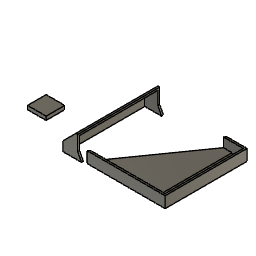
newest fin air guid v5 (Autodesk Fusion 360 design; units mm, degrees)
Autodesk Fusion 360 part; units mm, degrees
sketch "Sketch1" plane through (0, 0, 0) normal (0, 0, 1) x (1, 0, 0)
  line L0 (0, 0) -> (42, 0)
  line L1 (42, 0) -> (42, 44)
  line L2 (42, 44) -> (31, 44)
  line L3 (31, 44) -> (0, 0)
  dimension "d1" = 42
  dimension "d2" = 44
  dimension "d3" = 11
  constraint coincident L0.start L3.end
  constraint horizontal L0
  constraint perpendicular L0 L1
  constraint perpendicular L1 L2
  measures "d1" distance of L0.start L0.end
  measures "d2" distance of L0.end L1.end
  measures "d3" distance of L1.end L2.end
extrude "Extrude1" add sketch "Sketch1" along normal blind 6 makes body 1
sketch "Sketch2" plane through (42, 0, 0) normal (1, 0, 0) x (0, 1, 0)
  line L0 (0, 0) -> (44, 0)
  line L1 (44, 0) -> (44, 6)
  line L2 (44, 6) -> (0, 6)
  line L3 (0, 6) -> (0, 0)
  line L4 (1, 5) -> (43, 5)
  line L5 (43, 5) -> (43, 0)
  line L6 (43, 0) -> (1, 0)
  line L7 (1, 0) -> (1, 5)
  constraint horizontal L4
  constraint vertical L5
  constraint horizontal L6
  constraint vertical L7
  constraint coincident L0 L5.end
extrude "Extrude2" cut sketch "Sketch2" against normal blind 70 contours L0 L4 L5 L6 L7 bodies 1
sketch "Sketch3" plane through (0, 0, 5) normal (0, 0, -1) x (1, 0, 0)
  line L0 (0.7045, -1) -> (30.2955, -43)
  line L1 (30.2955, -43) -> (42, -43)
  line L2 (42, -43) -> (42, -1)
  line L3 (42, -1) -> (0.7045, -1)
  line L4 (42, -43) -> (41, -43)
  line L5 (41, -43) -> (41, -1)
  line L6 (41, -1) -> (42, -1)
  line L7 (42, -1) -> (42, -43)
  constraint horizontal L4
  constraint vertical L5
  constraint horizontal L6
  constraint vertical L7
  constraint coincident L3 L5.end
  constraint coincident L1.end L2.start
extrude "Extrude3" add sketch "Sketch3" along normal blind 5 contours L1 L2 L3 L4 L5 L6 L7 bodies 1
sketch "Sketch4" plane through (0, 0, 5) normal (0, 0, -1) x (1, 0, 0)
  line L0 (41, -43) -> (41, -1)
  line L1 (41, -1) -> (0.7045, -1)
  line L2 (0.7045, -1) -> (30.2955, -43)
  line L3 (30.2955, -43) -> (41, -43)
  line L4 (41, -43) -> (35, -43)
  line L5 (35, -43) -> (35, -1)
  line L6 (35, -1) -> (41, -1)
  line L7 (41, -1) -> (41, -43)
  dimension "d10" = 6
  dimension "d11" = 42
  constraint horizontal L4
  constraint vertical L5
  constraint horizontal L6
  constraint vertical L7
  constraint coincident L0.start L3.end
  measures "d10" distance of L0.start L4.end
  measures "d11" distance of L0.start L0.end
extrude "Extrude4" cut sketch "Sketch4" against normal blind 1 contours L0 L1 L3 L4 L5 L6 L7 bodies 1
sketch "Sketch5" plane through (0, 0, 0) normal (0, 0, 1) x (1, 0, 0)
  line L0 (-5, 0) -> (-13, 0)
  line L1 (-13, 0) -> (-13, 44)
  line L2 (-13, 44) -> (-5, 44)
  line L3 (-5, 44) -> (-5, 0)
  dimension "d14" = 8
  dimension "d15" = 44
  constraint horizontal L0
  constraint vertical L1
  constraint horizontal L2
  constraint vertical L3
  measures "d14" distance of L0.start L0.end
  measures "d15" distance of L0.start L2.end
extrude "Extrude5" add sketch "Sketch5" along normal blind 6 separate body makes body 2
extrude "Extrude6" add 1 faces at (-7.6667, 14.6667, 6) along direction (0, 0, 1) blind 2 on bodies 2 bodies 2
sketch "Sketch6" plane through (0, 44, 0) normal (0, 1, 0) x (-1, 0, 0)
  line L0 (5, 0) -> (13, 0)
  line L1 (13, 0) -> (13, 8)
  line L2 (13, 8) -> (5, 8)
  line L3 (5, 8) -> (5, 0)
  line L4 (5, 7) -> (12, 0)
  constraint coincident L3 L4.start
  constraint coincident L0 L4.end
extrude "Extrude7" cut sketch "Sketch6" against normal blind 53 contours L0 L3 L4 bodies 2
chamfer "Chamfer1" distance 7 angle 45 1 edges at (-13, 22, 8) on bodies 2
extrude "Extrude8" add 1 faces at (-12.6667, 14.6667, 0) along direction (0, 0, -1) blind 1 on bodies 2 bodies 2
extrude "Extrude9" add 1 faces at (-12, 29.3333, -0.3333) along direction (1, 0, 0) blind 7 on bodies 2 bodies 2
sketch "Sketch7" plane through (0, 0, 0) normal (0, 0, 1) x (-1, 0, 0)
  line L0 (12, -44) -> (12, 0)
  line L1 (12, 0) -> (5, 0)
  line L2 (5, 0) -> (5, -44)
  line L3 (5, -44) -> (12, -44)
  line L4 (5, -44) -> (12, -44)
  line L5 (12, -44) -> (12, -43)
  line L6 (12, -43) -> (5, -43)
  line L7 (5, -43) -> (5, -44)
  constraint horizontal L4
  constraint vertical L5
  constraint horizontal L6
  constraint vertical L7
  constraint coincident L0 L5.end
  constraint coincident L2.end L3.start
extrude "Extrude10" cut sketch "Sketch7" against normal blind 0.5 contours L0 L2 L3 L4 L5 L6 L7 bodies 2
extrude "Extrude11" cut 1 faces at (-9.6667, 43.6667, -0.5) along direction (0, 0, 1) blind 8.5 on bodies 2 bodies 2
extrude "Extrude12" add 1 faces at (-9.6667, 43.6667, -0.5) along direction (0, 0, 1) blind 8.5 on bodies 2 bodies 2
extrude "Extrude13" cut 1 faces at (-10, 43, 6) along direction (0, 1, 0) blind 1 on bodies 2 bodies 2
sketch "Sketch8" plane through (0, 0, 0) normal (0, 0, 1) x (-1, 0, 0)
  line L0 (5, -43) -> (12, -43)
  line L1 (12, -43) -> (12, 0)
  line L2 (12, 0) -> (5, 0)
  line L3 (5, 0) -> (5, -43)
  line L4 (5, 0) -> (12, 0)
  line L5 (12, 0) -> (12, -1)
  line L6 (12, -1) -> (5, -1)
  line L7 (5, -1) -> (5, 0)
  constraint horizontal L4
  constraint vertical L5
  constraint horizontal L6
  constraint vertical L7
  constraint coincident L1 L5.end
  constraint coincident L2.end L3.start
extrude "Extrude14" cut sketch "Sketch8" against normal blind 0.5 contours L1 L2 L3 L4 L5 L6 L7 bodies 2
extrude "Extrude15" cut 1 faces at (-7.3333, 0.3333, -0.5) along direction (0, 0, 1) blind 8.5 on bodies 2 bodies 2
extrude "Extrude16" add 1 faces at (-7.3333, 0.3333, -0.5) along direction (0, 0, 1) blind 8.5 on bodies 2 bodies 2
extrude "Extrude17" cut 1 faces at (-10, 1, 6) along direction (0, -1, 0) blind 1 on bodies 2 bodies 2
extrude "Extrude18" cut 1 faces at (-9.6667, 29, 0) along direction (0, 0, -1) blind 1 on bodies 2 bodies 2
extrude "Extrude19" add 1 faces at (-12.6667, 29, -1) along direction (0, 0, -1) blind 3 on bodies 2 bodies 2
move_body "Move1" bodies 1 to x (1, 0, 0) y (0, -1, 0) z (0, 0, -1) at (0, 50.0537, 12)
move_body "Move2" bodies 2 to x (1, 0, 0) y (0, 1, 0) z (0, 0, 1) at (0, 0, 3)
move_body "Move3" bodies 1 to x (1, 0, 0) y (0, 1, 0) z (0, 0, 1) at (0, 0, -7)
sketch "Sketch9" plane through (0, 0, 0) normal (0, 0, 1) x (1, 0, 0)
  line L0 (10, 10) -> (0, 10)
  line L1 (0, 10) -> (0, 20)
  line L2 (0, 20) -> (10, 20)
  line L3 (10, 20) -> (10, 10)
  constraint horizontal L0
  constraint vertical L1
  constraint horizontal L2
  constraint vertical L3
extrude "Extrude20" add sketch "Sketch9" along normal blind 2 separate body makes body 3
move_body "Move4" bodies 3 to x (1, 0, 0) y (0, 1, 0) z (0, 0, 1) at (0, 0, -1)
mirror "Mirror1" about plane through (0, 0, 0) normal (0, 1, 0) of bodies 1 makes body 4
move_body "Move5" bodies 3 to x (1, 0, 0) y (0, 1, 0) z (0, 0, 1) at (-42, 0, 0)
extrude "Extrude21" cut 1 faces at (14, 50.0537, 3) along direction (0, -1, 0) blind 47 on bodies 1 bodies 1
move_body "Move6" bodies 4 to x (1, 0, 0) y (0, 1, 0) z (0, 0, 1) at (-1, 51, 0)
sketch "Sketch10" plane through (0, 0, 0) normal (0, -1, 0) x (1, 0, 0)
  line L0 (-6, 11) -> (-13, 4)
  line L1 (-13, 4) -> (-13, -1)
  line L2 (-13, -1) -> (-5, -1)
  line L3 (-5, -1) -> (-5, 11)
  line L4 (-5, 11) -> (-6, 11)
  line L5 (-5, -1) -> (-3, -1)
  line L6 (-3, -1) -> (-5, 3)
  line L7 (-5, 3) -> (-5, -1)
  constraint coincident L2.end L3.start
  constraint perpendicular L3 L5
  constraint coincident L3 L6.end
extrude "Extrude22" add sketch "Sketch10" against normal blind 1 contours L3 L5 L6 L7 bodies 1 2
sketch "Sketch11" plane through (0, 44, 0) normal (0, 1, 0) x (-1, 0, 0)
  line L0 (13, 4) -> (6, 11)
  line L1 (6, 11) -> (5, 11)
  line L2 (5, 11) -> (5, -1)
  line L3 (5, -1) -> (13, -1)
  line L4 (13, -1) -> (13, 4)
  line L5 (5, -1) -> (3, -1)
  line L6 (3, -1) -> (5, 3)
  line L7 (5, -1) -> (5, 3)
  constraint coincident L2.end L3.start
  constraint perpendicular L2 L5
  constraint coincident L2 L6.end
extrude "Extrude23" add sketch "Sketch11" against normal blind 1 contours L2 L5 L6 L7 bodies 1
